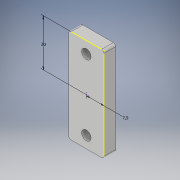
# Autodesk Inventor part: halter_test
Saved by Autodesk Inventor 2017 (Build 210142000, 142)
## iProperties
Part Number: halter_test
Material: Generisch
Document SubType Name: Modeling
Designer: Fabio
Density: 1 g/cm^3
Appearance: Vorgabe
Author: Fabio
Autodesk Inventor part; units mm, degrees
ref_plane "YZ Plane" through (0, 0, 0) normal (1, 0, 0) x (0, 1, 0)
ref_plane "XZ Plane" through (0, 0, 0) normal (0, 1, 0) x (-1, 0, 0)
ref_plane "XY Plane" through (0, 0, 0) normal (0, 0, 1) x (1, 0, 0)
sketch "Skizze1" plane through (0, 0, 0) normal (0, 1, 0) x (-1, 0, 0)
  line L0 (0, 0) -> (15, 0)
  line L1 (15, 0) -> (15, -40)
  line L2 (15, -40) -> (0, -40)
  line L3 (0, -40) -> (0, 0)
  dimension "d0" = 15
  dimension "d1" = 40
  constraints: 8 end point, 2 parallel, 1 horizontal, 1 perpendicular
  measures "d0" distance of L1.end L2.end
  measures "d1" distance of L0.end L1.end
extrude "Extrusion1" add sketch "Skizze1" along normal blind 5
fillet "Rundung1" radius 1 4 edges at (-15, 2.5, 0) (0, 2.5, 0) (0, 2.5, -40) (-15, 2.5, -40)
sketch "Skizze2" plane through (0, 0, 0) normal (0, -1, 0) x (1, 0, 0)
  line L0 (-1, 0) -> (-14, 0) projected
  line L1 (0, -39) -> (0, -1) projected
  line L2 (-14, -40) -> (-1, -40) projected
  point P0 (0, 0)
  point P1 (-7.5, -5)
  point P2 (-7.5, -35)
  dimension "d5" = 5
  dimension "d6" = 5
  dimension "d7" = 7.5
  dimension "d8" = 7.5
  dimension "d9" = 30
  measures "d5" distance from line of point (-7.5, -5) L0
  measures "d6" distance from line of point (-7.5, -35) L2
  measures "d7" distance from line of L1 point (-7.5, -5)
  measures "d8" distance from line of L1 point (-7.5, -35)
  measures "d9" distance of point (-7.5, -35) point (-7.5, -5)
hole "Bohrung1" at (-7.5, 0, -5) at (-7.5, 0, -35) direction (0, 1, 0) diameter 4 end through all
sketch "Skizze3" plane through (0, 0, 0) normal (0, -1, 0) x (1, 0, 0)
  line L0 (-1, 0) -> (-14, 0) projected
  line L1 (0, -39) -> (0, -1) projected
  point P0 (0, 0)
  point P1 (-7.5, -20)
  dimension "d17" = 20
  dimension "d18" = 7.5
  measures "d17" distance from line of L0 point (-7.5, -20)
  measures "d18" distance from line of L1 point (-7.5, -20)
